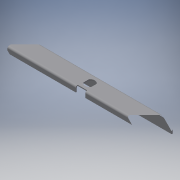
# Autodesk Inventor part: Part118
Saved by Autodesk Inventor 2016 (Build 200138000, 138)
## iProperties
Created: 2018-11-16
Part Number: Part118
Material: Generic
Document SubType Name: Sheet Metal
Designer: hovm
Density: 1 g/cm^3
Sheet Metal Rule: Default_mm
Appearance: Default
Author: hovm
Autodesk Inventor part; units mm, degrees
ref_plane "YZ Plane" through (0, 0, 0) normal (1, 0, 0) x (0, 1, 0)
ref_plane "XZ Plane" through (0, 0, 0) normal (0, 1, 0) x (-1, 0, 0)
ref_plane "XY Plane" through (0, 0, 0) normal (0, 0, 1) x (1, 0, 0)
sketch "Sketch1" plane through (0, 0, 0) normal (0, 0, 1) x (1, 0, 0)
  line L0 (0, 0) -> (310, 0)
  line L1 (310, 0) -> (310, 40)
  line L2 (310, 40) -> (0, 40)
  line L3 (0, 40) -> (0, 0)
  dimension "d1" = 40
  dimension "d2" = 310
  measures "d1" distance of L0.end L1.end
  measures "d2" distance of L1.end L2.end
extrude "Plate1" add sketch "Sketch1" along normal blind 2
sketch "Sketch2" plane through (310, 38, 2) normal (0, 1, 0) x (-1, 0, 0)
  line L0 (310, 0) -> (0, 0)
  line L1 (0, 0) -> (0, -25)
  line L2 (0, -25) -> (310, -25)
  line L3 (310, -25) -> (310, 0)
  constraints: 6 end point, 1 horizontal, 1 perpendicular, 1 vertical
edge flange "Flange1" height 25 angle 90 thickness 2 bend radius 2 thickness toward (0, 1, 0) relief tear relief width 2 relief depth 1 edges at (155, 40, 0) wall of the first edge with corners at (0, 38, 2) (310, 38, 2) (310, 38, -23) (0, 38, -23)
bend "Bend1"
corner "Corner1"
sketch "Sketch3" plane through (0, 2, 2) normal (0, -1, 0) x (1, 0, 0)
  line L0 (310, 0) -> (0, 0)
  line L1 (0, 0) -> (0, -12)
  line L2 (0, -12) -> (310, -12)
  line L3 (310, -12) -> (310, 0)
  constraints: 6 end point, 1 horizontal, 1 perpendicular, 1 vertical
edge flange "Flange2" height 12 angle 90 thickness 2 bend radius 2 thickness toward (0, -1, 0) relief tear relief width 2 relief depth 1 edges at (155, 0, 0) wall of the first edge with corners at (310, 2, 2) (0, 2, 2) (0, 2, -10) (310, 2, -10)
bend "Bend2"
corner "Corner2"
sketch "Sketch4" plane through (0, 0, 2) normal (0, 0, 1) x (1, 0, 0)
  arc A0 (146.75, 13.9172) -> (163.25, 13.9172) centre (155, 20) ccw
  line L0 (0, 4) -> (0, 36) projected
  line L1 (0, 40) -> (310, 40) projected
  line L2 (146.75, 26.0828) -> (146.75, 13.9172)
  line L3 (163.25, 26.0828) -> (163.25, 13.9172)
  arc A1 (146.75, 26.0828) -> (146.75, 13.9172) centre (155, 20) ccw construction
  arc A2 (163.25, 26.0828) -> (146.75, 26.0828) centre (155, 20) ccw
  arc A3 (163.25, 13.9172) -> (163.25, 26.0828) centre (155, 20) ccw construction
  point P0 (0, 0)
  point P1 (0, 20)
  point P2 (155, 40)
  dimension "d25" = 20.5
  dimension "d26" = 16.5
  constraints: 9 point on circle, 4 centre point, 4 end point, 2 horizontal alignment, 2 midpoint, 1 parallel, 1 vertical, 1 vertical alignment
  measures "d25" diameter of A0
  measures "d26" distance between parallel lines of L3 L2
extrude "Cut1" cut sketch "Sketch4" against normal blind 2
sketch "Sketch5" plane through (0, 0, 2) normal (0, 0, 1) x (1, 0, 0)
  line L0 (310, 4) -> (0, 4) projected
  line L1 (145, 4) -> (165, 4)
  line L2 (165, 4) -> (165, -2)
  line L3 (165, -2) -> (145, -2)
  line L4 (145, -2) -> (145, 4)
  point P0 (0, 0)
  point P1 (155, -2)
  point P2 (155, 4)
  dimension "d27" = 20
  dimension "d28" = 6
  constraints: 8 end point, 2 midpoint, 2 parallel, 1 horizontal, 1 perpendicular, 1 point on line, 1 vertical alignment
  measures "d27" distance of L2.end L3.end
  measures "d28" distance of L1.end L2.end
extrude "Cut2" cut sketch "Sketch5" against normal through all
equation "\"d23\" = Thickness"
equation "\"d29\" = Thickness"
equation "\"d3\" = BendReliefWidth"
equation "\"d4\" = BendReliefDepth"
equation "\"d5\" = MinimumRemnant"
equation "\"d6\" = BendRadius"
equation "\"d9\" = BendRadius"
equation "\"d10\" = CornerReliefSize"
equation "\"d11\" = GapSize"
equation "\"d12\" = JacobiRadiusSize"
equation "\"d13\" = BendReliefWidth"
equation "\"d14\" = BendReliefDepth"
equation "\"d15\" = MinimumRemnant"
equation "\"d16\" = BendRadius"
equation "\"d19\" = BendRadius"
equation "\"d20\" = CornerReliefSize"
equation "\"d21\" = GapSize"
equation "\"d22\" = JacobiRadiusSize"
equation "\"BendRadius\" = Thickness"
equation "\"BendReliefWidth\" = Thickness"
equation "\"BendReliefDepth\" = 0.5 * Thickness"
equation "\"CornerReliefSize\" = 4 * Thickness"
equation "\"MinimumRemnant\" = 2 * Thickness"
equation "\"TransitionRadius\" = BendRadius"
equation "\"JacobiRadiusSize\" = BendRadius"
equation "\"GapSize\" = Thickness"
equation "\"d0\" = BendRadius"
equation "\"Thickness\" = 2"
body "Solid1"
